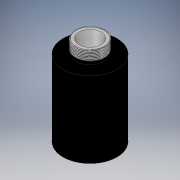
# Autodesk Inventor part: HPSt 15014-102 VS22
Saved by Autodesk Inventor 2017 (Build 210142000, 142)
## iProperties
Created: 2016-06-16
Part Number: HPSt 15014-102 VS22
Material: Generic
Document SubType Name: Modeling
Designer: Anna
Density: 1 g/cm^3
Appearance: Default
Author: Anna
Autodesk Inventor part; units mm, degrees
ref_plane "YZ Plane" through (0, 0, 0) normal (1, 0, 0) x (0, 1, 0)
ref_plane "XZ Plane" through (0, 0, 0) normal (0, 1, 0) x (-1, 0, 0)
ref_plane "XY Plane" through (0, 0, 0) normal (0, 0, 1) x (1, 0, 0)
sketch "Sketch1" plane through (0, 0, 0) normal (0, 1, 0) x (-1, 0, 0)
  circle A0 centre (0, 0) radius 11
  circle A1 centre (0, 0) radius 4.5
  dimension "d0" = 22
  dimension "d1" = 9
  constraints: 2 centre point, 2 coincident
  measures "d0" diameter of A0
  measures "d1" diameter of A1
extrude "Extrusion1" add sketch "Sketch1" along normal blind 25
sketch "Sketch3" plane through (0, 0, 0) normal (0, -1, 0) x (1, 0, 0)
  circle A0 centre (0, 0) radius 11
  circle A1 centre (0, 0) radius 6
  dimension "d5" = 22
  dimension "d6" = 12
  constraints: 2 centre point, 2 coincident
  measures "d5" diameter of A0
  measures "d6" diameter of A1
extrude "Extrusion2" add sketch "Sketch3" along normal blind 6
sketch "Sketch6" plane through (0, 25, 0) normal (0, 1, 0) x (1, 0, 0)
  circle A0 centre (0, 0) radius 4.5
  circle A1 centre (0, 0) radius 5.5
  dimension "d29" = 9
  dimension "d30" = 11
  constraints: 2 centre point, 2 coincident
  measures "d29" diameter of A0
  measures "d30" diameter of A1
extrude "Extrusion3" add sketch "Sketch6" along normal blind 1.5
sketch "Sketch7" plane through (0, 26.5, 0) normal (0, 1, 0) x (1, 0, 0)
  circle A0 centre (0, 0) radius 6
  circle A1 centre (0, 0) radius 4.5
  dimension "d33" = 12
  dimension "d34" = 9
  constraints: 2 centre point, 2 coincident
  measures "d33" diameter of A0
  measures "d34" diameter of A1
extrude "Extrusion4" add sketch "Sketch7" along normal blind 4
sketch "Sketch9" plane through (0, 30.5, 0) normal (1, 0, 0) x (0, 0, 1)
  line L0 (6, 0) -> (6, 4)
  line L1 (6, 4) -> (5.6737, 4)
  line L2 (5.6737, 4) -> (5.6737, 0)
  line L3 (5.6737, 0) -> (6, 0)
  line L4 (0, -7.9599) -> (0, 43.91) projected
  constraints: 8 end point
revolve "Revolution2" cut sketch "Sketch9" angle 360 about axis through (0, 30.5, 0) along (0, -1, 0)
sketch "Sketch10" plane through (0, 30.5, 0) normal (1, 0, 0) x (0, 0, 1)
  line L0 (6, 0) -> (6, 4)
  line L1 (6, 4) -> (5.6737, 4)
  line L2 (5.6737, 4) -> (5.6737, 0)
  line L3 (5.6737, 0) -> (6, 0)
  line L4 (0, -7.9599) -> (0, 43.91) projected
  constraints: 8 end point
revolve "Revolution3" add sketch "Sketch10" angle 360 about axis through (0, 30.5, 0) along (0, -1, 0) separate body
sketch "Sketch8" plane through (0, 30.5, 0) normal (-1, 0, 0) x (0, -1, 0)
  line L0 (-0.2963, -5.7006) -> (-0.2501, -5.7006) construction
  line L1 (0.0461, -5.9735) -> (-0.0001, -6.0535) construction
  line L2 (-0.5001, -6.0535) -> (-0.5463, -5.9735) construction
  line L3 (-0.2039, -5.7006) -> (-0.2501, -5.6205) construction
  line L4 (-0.2501, -5.6205) -> (-0.2963, -5.7006) construction
  line L5 (-0.5001, -6.0535) -> (-0.4539, -5.9735) construction
  line L6 (-0.2039, -5.7006) -> (-0.0463, -5.9735)
  line L7 (-0.5463, -5.9735) -> (-0.4539, -5.9735) construction
  arc A0 (-0.5463, -5.9735) -> (-0.5001, -6.0002) centre (-0.5001, -5.9468) ccw construction
  line L8 (0.0461, -5.9735) -> (-0.0463, -5.9735) construction
  line L9 (-0.5001, -6.0535) -> (-0.5001, -5.9735) construction
  line L10 (-0.0001, -6.0535) -> (-0.0001, -5.9735) construction
  line L11 (-0.2501, -5.6205) -> (-0.2501, -5.6739) construction
  line L12 (-0.5001, -6.0002) -> (-0.0001, -6.0002)
  arc A1 (-0.5001, -6.0002) -> (-0.4539, -5.9735) centre (-0.5001, -5.9468) ccw
  line L13 (-0.0463, -5.9735) -> (-0.0001, -6.0535) construction
  line L14 (-0.4539, -5.9735) -> (-0.2963, -5.7006)
  line L15 (-0.0001, -0.0002) -> (-0.0001, 0.0177)
  line L16 (-0.0001, 0.0177) -> (-0.0001, -0.0002)
  line L17 (-0.0001, -0.0002) -> (0.0334, -0.0002)
  arc A2 (-0.0463, -5.9735) -> (-0.0001, -6.0002) centre (-0.0001, -5.9468) ccw
  arc A3 (-0.0001, -6.0002) -> (0.0461, -5.9735) centre (-0.0001, -5.9468) ccw construction
  arc A4 (-0.2501, -5.6739) -> (-0.2963, -5.7006) centre (-0.2501, -5.7272) ccw
  arc A5 (-0.2039, -5.7006) -> (-0.2501, -5.6739) centre (-0.2501, -5.7272) ccw
  line L18 (-0.2501, -5.6739) -> (-0.2501, -5.7006) construction
  line L19 (-0.2501, -5.7006) -> (-0.2039, -5.7006) construction
  dimension "d41" = 60
  dimension "d42" = 0.08
  dimension "d43" = 0.08
  dimension "Sketch8_ThreadOffset" = 0
  dimension "Sketch8_MajorRadius" = 6
  dimension "d46" = 0.5
  dimension "Sketch8_MinorRadius" = 5.6737
  constraints: 40 end point, 12 point on circle, 10 parallel, 8 tangent, 6 centre point, 6 collinear, 2 midpoint, 2 point on line, 1 horizontal, 1 perpendicular, 3 other
  measures "d41" angle of L6 L14
  measures "d42" distance of L3.end L0.end
  measures "d43" distance of L1.end L10.end
  measures "Sketch8_ThreadOffset" distance between parallel lines of L15 L10
  measures "Sketch8_MajorRadius" distance from line of L12 L15.start
  measures "d46" distance from line of L1.end L9
  measures "Sketch8_MinorRadius" distance edge to line of A5 L17
coil "Coil2" sketch "Sketch8" operation cut axis through (0, 30.5, 0) along (0, -1, 0) pitch 0.5005 turns 9.99001 hand right bodies 2
sketch "Sketch12" plane through (0, -6, 0) normal (-1, 0, 0) x (0, 0, 1)
  line L0 (6, 0) -> (6, 6)
  line L1 (6, 6) -> (5.6737, 6)
  line L2 (5.6737, 6) -> (5.6737, 0)
  line L3 (5.6737, 0) -> (6, 0)
  line L4 (0, -7.9914) -> (0, 44.0991) projected
  constraints: 8 end point
revolve "Revolution4" add sketch "Sketch12" angle 360 about axis through (0, -6, 0) along (0, 1, 0) separate body
sketch "Sketch11" plane through (0, -6, 6) normal (1, 0, 0) x (0, 1, 0)
  line L0 (-0.2963, -0.0268) -> (-0.2501, -0.0268) construction
  line L1 (0.0461, -0.2998) -> (-0.0001, -0.3798) construction
  line L2 (-0.5001, -0.3798) -> (-0.5463, -0.2998) construction
  line L3 (-0.2039, -0.0268) -> (-0.2501, 0.0532) construction
  line L4 (-0.2501, 0.0532) -> (-0.2963, -0.0268) construction
  line L5 (-0.5001, -0.3798) -> (-0.4539, -0.2998) construction
  line L6 (-0.2039, -0.0268) -> (-0.0463, -0.2998)
  line L7 (-0.5463, -0.2998) -> (-0.4539, -0.2998) construction
  arc A0 (-0.5463, -0.2998) -> (-0.5001, -0.3265) centre (-0.5001, -0.2731) ccw construction
  line L8 (0.0461, -0.2998) -> (-0.0463, -0.2998) construction
  line L9 (-0.5001, -0.3798) -> (-0.5001, -0.2998) construction
  line L10 (-0.0001, -0.3798) -> (-0.0001, -0.2998) construction
  line L11 (-0.2501, 0.0532) -> (-0.2501, -0.0002) construction
  line L12 (-0.5001, -0.3265) -> (-0.0001, -0.3265)
  arc A1 (-0.5001, -0.3265) -> (-0.4539, -0.2998) centre (-0.5001, -0.2731) ccw
  line L13 (-0.0463, -0.2998) -> (-0.0001, -0.3798) construction
  line L14 (-0.4539, -0.2998) -> (-0.2963, -0.0268)
  line L15 (-0.0001, -0.0002) -> (-0.0001, 0.0177)
  line L16 (-0.0001, 0.0177) -> (-0.0001, -0.0002)
  line L17 (-0.0001, -0.0002) -> (0.0334, -0.0002)
  arc A2 (-0.0463, -0.2998) -> (-0.0001, -0.3265) centre (-0.0001, -0.2731) ccw
  arc A3 (-0.0001, -0.3265) -> (0.0461, -0.2998) centre (-0.0001, -0.2731) ccw construction
  arc A4 (-0.2501, -0.0002) -> (-0.2963, -0.0268) centre (-0.2501, -0.0535) ccw
  arc A5 (-0.2039, -0.0268) -> (-0.2501, -0.0002) centre (-0.2501, -0.0535) ccw
  line L18 (-0.2501, -0.0002) -> (-0.2501, -0.0268) construction
  line L19 (-0.2501, -0.0268) -> (-0.2039, -0.0268) construction
  dimension "d60" = 60
  dimension "d61" = 0.08
  dimension "d62" = 0.08
  dimension "Sketch11_ThreadOffset" = 0
  dimension "Sketch11_MajorRadius" = 0.3263
  dimension "d65" = 0.5
  dimension "Sketch11_MinorRadius" = 0
  constraints: 40 end point, 12 point on circle, 10 parallel, 8 tangent, 6 centre point, 6 collinear, 2 midpoint, 2 point on line, 1 horizontal, 1 perpendicular, 3 other
  measures "d60" angle of L6 L14
  measures "d61" distance of L3.end L0.end
  measures "d62" distance of L1.end L10.end
  measures "Sketch11_ThreadOffset" distance between parallel lines of L15 L10
  measures "Sketch11_MajorRadius" distance from line of L12 L15.start
  measures "d65" distance from line of L1.end L9
  measures "Sketch11_MinorRadius" distance edge to line of A5 L17
coil "Coil3" sketch "Sketch11" operation cut axis through (0, -6, 0) along (0, 1, 0) pitch 0.5005 turns 13.986014 hand right bodies 3
sketch "Sketch23" plane through (0, -6, 0) normal (0, -1, 0) x (1, 0, 0)
  point P0 (0, 7.5)
  point P1 (-7.5, 0)
  point P2 (0, -7.5)
hole "Hole6" at (0, -6, 7.5) direction (0, 1, 0) diameter 2 depth 4 tip angle 118 bodies 1
sketch "Sketch24" plane through (0, -6, 0) normal (0, -1, 0) x (1, 0, 0)
  point P0 (0, 7.5)
  point P1 (-7.5, 0)
  point P2 (0, -7.5)
  point P3 (7.5, 0)
hole "Hole7" at (0, -6, 7.5) at (-7.5, -6, 0) at (0, -6, -7.5) at (7.5, -6, 0) direction (0, 1, 0) diameter 2 depth 4 tip angle 118 bodies 1
thread "Thread8" size "M2x0.25" class "6H" standard "ISO Metric profile" full length
thread "Thread9" size "M2x0.25" class "6H" standard "ISO Metric profile" full length
thread "Thread10" size "M2x0.25" class "6H" standard "ISO Metric profile" full length
thread "Thread11" size "M2x0.25" class "6H" standard "ISO Metric profile" full length
equation "\"d41\" = d48"
equation "\"d42\" = 0.160083 * Sketch8_Pitch"
equation "\"d43\" = 0.160083 * Sketch8_Pitch"
equation "\"d46\" = Sketch8_Pitch"
equation "\"d60\" = d67"
equation "\"d61\" = 0.160083 * Sketch11_Pitch"
equation "\"d62\" = 0.160083 * Sketch11_Pitch"
equation "\"d65\" = Sketch11_Pitch"
equation "\"d18\" = 60deg"
equation "\"Sketch4_Pitch\" = 0.75"
equation "\"d48\" = 60deg"
equation "\"Sketch8_Pitch\" = 0.5"
equation "\"d67\" = 60deg"
equation "\"Sketch11_Pitch\" = 0.5"
equation "\"d108\" = 60deg"
equation "\"Sketch14_Pitch\" = 0.4"
equation "\"d126\" = 60deg"
equation "\"Sketch16_Pitch\" = 0.4"
equation "\"d144\" = 60deg"
equation "\"Sketch18_Pitch\" = 0.4"
equation "\"d162\" = 60deg"
equation "\"Sketch20_Pitch\" = 0.4"
body "Solid1"
body "Solid3"
body "Solid4"
